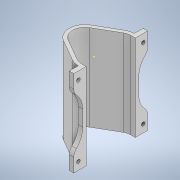
# Autodesk Inventor part: battery_1
Saved by Autodesk Inventor 2020 (Build 240168000, 168)
## iProperties
Created: 2022-07-15
Part Number: battery_1
Material: Типовые
Document SubType Name: Modeling
Designer: akapu
Density: 1 g/cm^3
Appearance: По умолчанию
Author: akapu
Autodesk Inventor part; units mm, degrees
ref_plane "YZ Plane" through (0, 0, 0) normal (1, 0, 0) x (0, 1, 0)
ref_plane "XZ Plane" through (0, 0, 0) normal (0, 1, 0) x (-1, 0, 0)
ref_plane "XY Plane" through (0, 0, 0) normal (0, 0, 1) x (1, 0, 0)
sketch "Эскиз1" plane through (0, 0, 0) normal (0, 1, 0) x (-1, 0, 0)
  circle A0 centre (0, 0) radius 11
  circle A1 centre (0, -22) radius 11
  circle A2 centre (19.0526, -11) radius 11
  line L0 (0, 0) -> (7, 12.1244)
  line L1 (0, 0) -> (14, 0) construction
  line L2 (0, -22) -> (7, -34.1244)
  line L3 (0, -22) -> (14, -22) construction
  line L4 (5.5, 9.5263) -> (24.5526, -1.4737)
  line L5 (5.5, -31.5263) -> (24.5526, -20.5263)
  circle A3 centre (0, 0) radius 14
  circle A4 centre (0, -22) radius 14
  circle A5 centre (19.0526, -11) radius 14
  line L6 (7, 12.1244) -> (26.0526, 1.1244)
  line L7 (7, -34.1244) -> (26.0526, -23.1244)
  line L8 (-14, 0) -> (-9, 0)
  line L9 (0, 11) -> (8.6603, 11) construction
  line L10 (0, 14) -> (-9, 14)
  line L11 (0, 11) -> (-9, 11)
  line L12 (0, -36) -> (-9, -36)
  line L13 (0, -33) -> (-9, -33)
  line L14 (-9, -36) -> (-9, 14)
  line L15 (-9, 11) -> (-6, 11)
  line L16 (-6, 11) -> (-6, 22)
  line L17 (-6, 22) -> (-9, 22)
  line L18 (-9, 22) -> (-9, 11)
  line L19 (-9, -33) -> (-6, -33)
  line L20 (-6, -33) -> (-6, -44)
  line L21 (-6, -44) -> (-9, -44)
  line L22 (-9, -44) -> (-9, -33)
  line L23 (-9, 11) -> (-4, 11)
  line L24 (-4, 11) -> (0, 11)
  line L25 (0, 11) -> (0, 22)
  line L26 (0, 22) -> (-4, 22)
  line L27 (-4, 22) -> (-4, 11)
  line L28 (-9, -33) -> (-4, -33)
  line L29 (-4, -33) -> (0, -33)
  line L30 (0, -33) -> (0, -44)
  line L31 (0, -44) -> (-4, -44)
  line L32 (-4, -44) -> (-4, -33)
  line L33 (-4, 11) -> (-4, -36)
  point P0 (-6, -36)
  point P1 (-6, 14)
  dimension "d10" = 22
  dimension "d12" = 22
  dimension "d13" = 14
  dimension "d14" = 60
  dimension "d15" = 14
  dimension "d16" = 60
  dimension "d17" = 28
  dimension "d20" = 9
  dimension "d21" = 3
  dimension "d22" = 11
  dimension "d23" = 3
  dimension "d24" = 11
  dimension "d53" = 5
  dimension "d54" = 4
  dimension "d55" = 5
  constraints: 68 end point, 14 point on circle, 9 horizontal, 9 parallel, 9 tangent, 7 perpendicular, 6 centre point, 6 point on line, 3 coincident, 2 equal length, 1 vertical
  measures "d10" diameter of A0
  measures "d12" diameter of A1
  measures "d13" distance of L0.start L0.end
  measures "d14" angle of L1 L0
  measures "d15" distance of L2.start L2.end
  measures "d16" angle of L2 L3
  measures "d17" diameter of A5
  measures "d20" distance of L13.start L13.end
  measures "d21" distance of L17.end L16.end
  measures "d22" distance of L16.end L15.end
  measures "d23" distance of L20.end L21.end
  measures "d24" distance of L19.end L20.end
  measures "d53" distance of L11.end L23.end
  measures "d54" distance of L26.end L25.end
  measures "d55" distance of L13.end L28.end
extrude "Выдавливание1" add sketch "Эскиз1" along normal blind 77 contours A0 L25 A3 L0 | L0 A3 L4 | L11 L27 A3 L25 | L6 A5 L4 A3 | A3 L27 L10 | L10 L27 L26 L25 | A5 L5 A2 L4 | L7 A4 L5 A5 | A4 L30 A1 L2 | L2 L5 A4 | L12 L32 A4 | L30 L31 L32 L12 | A4 L32 L13 L30
sketch "Эскиз6" plane through (4, 0, -33) normal (1, 0, 0) x (0, 0, -1)
  line L0 (11, 0) -> (11, 77) projected
  line L1 (11, 0) -> (11, 31.5)
  line L2 (11, 77) -> (11, 45.5)
  line L3 (-47, 0) -> (-55, 0) projected
  line L4 (-55, 0) -> (-55, 31.5)
  line L5 (-55, 0) -> (-55, 77) projected
  line L6 (-55, 77) -> (-55, 45.5)
  line L7 (-47, 0) -> (-47, 77) projected
  line L8 (-55, 45.5) -> (-47, 45.5)
  line L9 (-47, 45.5) -> (-47, 31.5)
  line L10 (-47, 31.5) -> (-55, 31.5)
  line L11 (-55, 31.5) -> (-55, 45.5)
  line L12 (3, 0) -> (3, 77) projected
  line L13 (11, 31.5) -> (3, 31.5)
  line L14 (3, 31.5) -> (3, 45.5)
  line L15 (3, 45.5) -> (11, 45.5)
  line L16 (11, 45.5) -> (11, 31.5)
  arc A0 (3, 31.5) -> (11, 15.75) centre (22.9984, 31.7512) ccw
  arc A1 (11, 61.25) -> (3, 45.5) centre (22.9984, 45.2488) ccw
  arc A2 (-47, 45.5) -> (-55, 61.25) centre (-66.9984, 45.2488) ccw
  arc A3 (-55, 15.75) -> (-47, 31.5) centre (-66.9984, 31.7512) ccw
  point P0 (-33, 0)
  point P1 (3, 31.5)
  point P2 (11, 15.75)
  dimension "d56" = 31.5
  dimension "d57" = 31.5
  dimension "d58" = 31.5
  dimension "d59" = 31.5
  dimension "d60" = 20
  dimension "d61" = 20
  dimension "d62" = 20
  dimension "d63" = 20
  constraints: 24 end point, 8 point on circle, 7 point on line, 4 centre point, 4 parallel, 3 midpoint, 2 horizontal, 2 perpendicular
  measures "d56" distance of L0.start L1.end
  measures "d57" distance of L0.end L2.end
  measures "d58" distance of L3.end L4.end
  measures "d59" distance of L5.end L6.end
  measures "d60" radius of A0
  measures "d61" radius of A1
  measures "d62" radius of A2
  measures "d63" radius of A3
extrude "Выдавливание5" cut sketch "Эскиз6" against normal blind 4 contours A0 L13 L0 | L13 L12 L15 L0 | L15 A1 L0 | L10 L5 L8 L7 | A3 L4 L10 | L8 L5 A2
fillet "Сопряжение2" radius 8 4 edges at (2, 15.75, -44) (2, 61.25, -44) (2, 61.25, 22) (2, 15.75, 22)
sketch "Эскиз7" plane through (0, 0, 14) normal (-1, 0, 0) x (0, 0, 1)
  line L0 (8, 0) -> (8, 12.1537) projected
  line L1 (8, 0) -> (4, 0)
  line L2 (8, 7) -> (8, 0)
  line L3 (4, 7) -> (-54, 7)
  line L4 (-54, 7) -> (-54, 70)
  line L5 (-54, 70) -> (4, 70)
  line L6 (4, 70) -> (4, 7)
  line L7 (4, 7) -> (1.4, 7)
  line L8 (-54, 70) -> (-51.4, 70)
  line L9 (1.4, 7) -> (-51.4, 7)
  line L10 (-51.4, 7) -> (-51.4, 70)
  line L11 (-51.4, 70) -> (1.4, 70)
  line L12 (1.4, 70) -> (1.4, 7)
  line L13 (1.4, 8.5011) -> (4, 10.0022)
  line L14 (4, 10.0022) -> (6.6, 8.5011)
  line L15 (6.6, 8.5011) -> (6.6, 5.4989)
  line L16 (6.6, 5.4989) -> (4, 3.9978)
  line L17 (4, 3.9978) -> (1.4, 5.4989)
  line L18 (1.4, 5.4989) -> (1.4, 8.5011)
  line L19 (-51.4, 5.4989) -> (-54, 3.9978)
  line L20 (-54, 3.9978) -> (-56.6, 5.4989)
  line L21 (-56.6, 5.4989) -> (-56.6, 8.5011)
  line L22 (-56.6, 8.5011) -> (-54, 10.0022)
  line L23 (-54, 10.0022) -> (-51.4, 8.5011)
  line L24 (-51.4, 8.5011) -> (-51.4, 5.4989)
  line L25 (-51.4, 68.4989) -> (-54, 66.9978)
  line L26 (-54, 66.9978) -> (-56.6, 68.4989)
  line L27 (-56.6, 68.4989) -> (-56.6, 71.5011)
  line L28 (-56.6, 71.5011) -> (-54, 73.0022)
  line L29 (-54, 73.0022) -> (-51.4, 71.5011)
  line L30 (-51.4, 71.5011) -> (-51.4, 68.4989)
  line L31 (1.4, 71.5011) -> (4, 73.0022)
  line L32 (4, 73.0022) -> (6.6, 71.5011)
  line L33 (6.6, 71.5011) -> (6.6, 68.4989)
  line L34 (6.6, 68.4989) -> (4, 66.9978)
  line L35 (4, 66.9978) -> (1.4, 68.4989)
  line L36 (1.4, 68.4989) -> (1.4, 71.5011)
  point P0 (-14, 0)
  point P1 (1.4, 68.4989)
  point P2 (1.4, 8.5011)
  dimension "d69" = 58
  dimension "d70" = 63
  dimension "d71" = 2.6
  dimension "d72" = 2.6
  constraints: 72 end point, 4 coincident, 4 midpoint, 4 parallel, 3 horizontal, 2 perpendicular, 2 point on line, 52 other
  measures "d69" distance of L4.end L5.end
  measures "d70" distance of L3.end L4.end
  measures "d71" distance of L3.start L7.end
  measures "d72" distance of L4.end L8.end
extrude "Выдавливание6" cut sketch "Эскиз7" against normal blind 2 contours L6 L14 L15 L16 L17 L18 L3 | L3 L12 L13 L6 | L24 L19 L20 L21 L22 L4 L3 | L3 L4 L23 L10 | L35 L12 L5 L6 | L6 L5 L36 L31 L32 L33 L34 | L25 L4 L5 L10 | L26 L27 L28 L29 L30 L5 L4
sketch "Эскиз8" plane through (2, 0, 14) normal (-1, 0, 0) x (0, 0, 1)
  line L0 (4, 7) -> (-54, 7)
  line L1 (-54, 7) -> (-54, 70)
  line L2 (-54, 70) -> (4, 70)
  line L3 (4, 70) -> (4, 7)
  circle A0 centre (4, 7) radius 1.6
  circle A1 centre (-54, 7) radius 1.6
  circle A2 centre (-54, 70) radius 1.6
  circle A3 centre (4, 70) radius 1.6
  point P0 (-14, 0)
  dimension "d75" = 3.2
  dimension "d76" = 3.2
  dimension "d77" = 3.2
  dimension "d78" = 3.2
  constraints: 8 end point, 4 centre point, 4 coincident, 2 parallel, 1 horizontal, 1 perpendicular
  measures "d75" diameter of A0
  measures "d76" diameter of A1
  measures "d77" diameter of A2
  measures "d78" diameter of A3
extrude "Выдавливание7" cut sketch "Эскиз8" against normal blind 2 contours A1 L1 L0 | L0 L1 A1 | A0 L3 L0 | L0 L3 A0 | A2 L2 L1 | L1 L2 A2 | A3 L2 L3 | L3 L2 A3
sketch "Эскиз9" plane through (0, 77, 0) normal (0, 1, 0) x (1, 0, 0)
  point P0 (0, 0)
